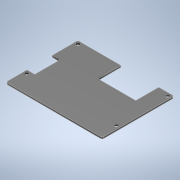
# Autodesk Inventor part: A203-V2-Expansion-Board
Saved by Autodesk Inventor 2022.3 (Build 263350000, 350)
## iProperties
Created: 2023-05-14
Part Number: A203-V2-Expansion-Board
Material: Generic
Document SubType Name: Modeling
Designer: Masato Kubotera
Density: 1 g/cm^3
Appearance: 滑らか - 黒
Author: Masato Kubotera
Autodesk Inventor part; units mm, degrees
ref_plane "YZ Plane" through (0, 0, 0) normal (1, 0, 0) x (0, 1, 0)
ref_plane "XZ Plane" through (0, 0, 0) normal (0, 1, 0) x (-1, 0, 0)
ref_plane "XY Plane" through (0, 0, 0) normal (0, 0, 1) x (1, 0, 0)
sketch "スケッチ1" plane through (0, 0, 0) normal (0, 0, 1) x (1, 0, 0)
  line L0 (32.5, 43.5) -> (-32.5, 43.5)
  line L1 (-32.5, 43.5) -> (-32.5, -43.5)
  line L2 (-32.5, -43.5) -> (32.5, -43.5)
  line L3 (32.5, -43.5) -> (32.5, 43.5)
  line L4 (32.5, 43.5) -> (-32.5, -43.5) construction
  line L5 (-32.5, 43.5) -> (32.5, -43.5) construction
  line L6 (-32.5, 29.7) -> (-11.7, 29.7)
  line L7 (-11.7, 29.7) -> (-11.7, -4.5)
  line L8 (-11.7, -4.5) -> (-32.5, -4.5)
  line L9 (-9.3, -43.5) -> (-9.3, -36.5)
  line L10 (-9.3, -36.5) -> (13.5, -36.5)
  line L11 (13.5, -36.5) -> (13.5, -43.5)
  line L12 (-29.7, -40.6) -> (16.7, -40.6) construction
  line L13 (16.7, -40.6) -> (16.7, 40.6) construction
  line L14 (16.7, 40.6) -> (-29.7, 40.6) construction
  line L15 (-29.7, 40.6) -> (-29.7, -40.6) construction
  line L16 (-29.7, -40.6) -> (16.7, 40.6) construction
  line L17 (16.7, -40.6) -> (-29.7, 40.6) construction
  circle A0 centre (16.7, 40.6) radius 1.6
  circle A1 centre (-29.7, 40.6) radius 1.6
  circle A2 centre (-29.7, -40.6) radius 1.6
  circle A3 centre (16.7, -40.6) radius 1.6
  line L18 (-32.5, 0) -> (32.5, 0) construction
  point P0 (0, 0)
  point P1 (0, 0)
  point P2 (0, 0)
  point P3 (-6.5, 0)
  dimension "d0" = 87
  dimension "d1" = 65
  dimension "d2" = 13.8
  dimension "d3" = 39
  dimension "d4" = 20.8
  dimension "d5" = 7
  dimension "d6" = 19
  dimension "d7" = 23.2
  dimension "d8" = 22.8
  dimension "d9" = 34.2
  dimension "d10" = 3.2
  dimension "d12" = 81.2
  dimension "d13" = 46.4
  dimension "d19" = 2.8
  constraints: 38 end point, 7 midpoint, 6 perpendicular, 5 point on line, 4 centre point, 4 coincident, 4 parallel, 3 equal radius, 3 horizontal, 1 vertical
  measures "d0" distance of L2.end L0.start
  measures "d1" distance of L0.start L0.end
  measures "d2" distance between parallel lines of L0 L6
  measures "d3" distance between parallel lines of L2 L8
  measures "d4" distance of L6.start L6.end
  measures "d5" distance of L10.end L11.end
  measures "d6" distance of L11.end L2.end
  measures "d7" distance of L1.end L9.start
  measures "d8" distance of L9.end L10.end
  measures "d9" distance of L6.end L7.end
  measures "d10" diameter of A0
  measures "d12" distance of L12.end L13.end
  measures "d13" distance of L13.end L14.end
  measures "d19" horizontal distance of L14.end L0.end
extrude "押し出し1" add sketch "スケッチ1" along normal blind 1.6 contours L3 L2 L11 L10 L9 L1 L8 L7 L6 L0
chamfer "面取り1" distance 1 angle 45 4 edges at (32.5, -43.5, 0.8) (-32.5, -43.5, 0.8) (32.5, 43.5, 0.8) (-32.5, 43.5, 0.8)
